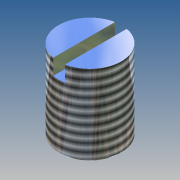
# Autodesk Inventor part: Terminal Screw
Saved by Autodesk Inventor 2014 (Build 180170000, 170)
## iProperties
Shininess: 64.0
Angle Display Precision: 2
Document Length Units: 11269
Document Angle Units: 11279
Document Time Units: 11290
Document Mass Units: 11283
Document Length Units Precision: 3
Document Angle Units Precision: 2
Created: 2003-03-14
Part Number: Terminal Screw
Material: Steel, Mild
Document SubType Name: Modeling
Designer: t8558es
Vendor: FCI Burndy
Density: 1 g/cm^3
Appearance: Chrome - Polished
Density: 0.0
Volumn: 0.0
Area: 0.0
PropertySet Name: Model Information
Control State: 0
Master: False
Checked Out: False
Author: t8558es
Autodesk Inventor part; units mm, degrees
ref_plane "YZ Plane" through (0, 0, 0) normal (1, 0, 0) x (0, 1, 0)
ref_plane "XZ Plane" through (0, 0, 0) normal (0, 1, 0) x (-1, 0, 0)
ref_plane "XY Plane" through (0, 0, 0) normal (0, 0, 1) x (1, 0, 0)
sketch "Sketch1" plane through (0, 0, 0) normal (0, 0, 1) x (1, 0, 0)
  circle A0 centre (0, 0) radius 4
  dimension "d0" = 8
  constraints: 1 centre point
  measures "d0" diameter of A0
extrude "Extrusion1" add sketch "Sketch1" along normal blind 10.3
chamfer "Chamfer1" distance 0.3 angle 45 1 edges at (-4, 0, 0)
thread "Thread1" size "M8x1" class "6g" standard "ANSI Metric M Profile" full length
sketch "Sketch2" plane through (0, 0, 10.3) normal (0, 0, 1) x (1, 0, 0)
  circle A0 centre (0, 0) radius 4 projected
  line L0 (-0.75, -3.9291) -> (-0.75, 3.9291)
  line L1 (0.75, -3.9291) -> (0.75, 3.9291)
  dimension "d7" = 1.5
  dimension "d8" = 0.75
  constraints: 4 end point, 4 point on circle, 1 parallel, 1 vertical
  measures "d7" distance between parallel lines of L1 L0
  measures "d8" distance from line of L0 A0.centre
extrude "Extrusion2" cut sketch "Sketch2" against normal blind 2 contours L1 A0 L0
equation "\"d8\" = 0.5 * d7"
body "Solid1"
